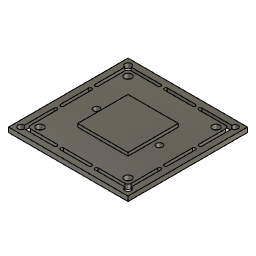
oat_guide_scope (Autodesk Fusion 360 archive; units mm, degrees)
design "ar0130"
Autodesk Fusion 360 part; units mm, degrees
sketch "Skizze1" plane through (0, 0, 0) normal (0, 0, 1) x (1, 0, 0)
  line L0 (-19, 19) -> (19, 19)
  line L1 (19, 19) -> (19, -19)
  line L2 (19, -19) -> (-19, -19)
  line L3 (-19, -19) -> (-19, 19)
  circle A0 centre (-14, 14) radius 1.175
  line L4 (0, 19) -> (0, -19) construction
  line L5 (-19, 0) -> (19, 0) construction
  circle A1 centre (14, 14) radius 1.175
  circle A2 centre (-14, -14) radius 1.175
  circle A3 centre (14, -14) radius 1.175
  circle A4 centre (-17, 17) radius 1
  circle A5 centre (17, 17) radius 1
  circle A6 centre (-17, -17) radius 1
  circle A7 centre (17, -17) radius 1
  circle A8 centre (-10, 0) radius 1
  circle A9 centre (10, 0) radius 1
  line L6 (-17, 16.5) -> (-6.5, 16.5) construction
  line L7 (-4.5, 16.5) -> (4.5, 16.5) construction
  line L8 (-4.5, 16) -> (4.5, 16)
  arc A10 (4.5, 16) -> (4.5, 17) centre (4.5, 16.5) ccw
  line L9 (4.5, 17) -> (-4.5, 17)
  arc A11 (-4.5, 17) -> (-4.5, 16) centre (-4.5, 16.5) ccw
  line L10 (-4.5, 16.5) -> (4.5, 16.5) construction
  line L11 (-6.5, 17) -> (-17, 17)
  arc A12 (-17, 17) -> (-17, 16) centre (-17, 16.5) ccw
  line L12 (-17, 16) -> (-6.5, 16)
  arc A13 (-6.5, 16) -> (-6.5, 17) centre (-6.5, 16.5) ccw
  line L13 (-6.5, 16.5) -> (-17, 16.5) construction
  line L14 (-19, 19) -> (19, -19) construction
  line L15 (6.5, 17) -> (17, 17)
  arc A14 (17, 16) -> (17, 17) centre (17, 16.5) ccw
  arc A15 (6.5, 17) -> (6.5, 16) centre (6.5, 16.5) ccw
  line L16 (17, 16) -> (6.5, 16)
  line L17 (-6.5, -17) -> (-17, -17)
  arc A16 (-17, -16) -> (-17, -17) centre (-17, -16.5) ccw
  arc A17 (-6.5, -17) -> (-6.5, -16) centre (-6.5, -16.5) ccw
  line L18 (4.5, -17) -> (-4.5, -17)
  arc A18 (-4.5, -16) -> (-4.5, -17) centre (-4.5, -16.5) ccw
  arc A19 (4.5, -17) -> (4.5, -16) centre (4.5, -16.5) ccw
  arc A20 (6.5, -16) -> (6.5, -17) centre (6.5, -16.5) ccw
  line L19 (6.5, -17) -> (17, -17)
  arc A21 (17, -17) -> (17, -16) centre (17, -16.5) ccw
  line L20 (17, -16) -> (6.5, -16)
  line L21 (-4.5, -16) -> (4.5, -16)
  line L22 (-17, -16) -> (-6.5, -16)
  line L23 (-17, -4.5) -> (-17, 4.5)
  arc A22 (-16, 4.5) -> (-17, 4.5) centre (-16.5, 4.5) ccw
  arc A23 (-17, -4.5) -> (-16, -4.5) centre (-16.5, -4.5) ccw
  line L24 (-16, 4.5) -> (-16, -4.5)
  arc A24 (17, 4.5) -> (16, 4.5) centre (16.5, 4.5) ccw
  line L25 (16, 4.5) -> (16, -4.5)
  arc A25 (16, -4.5) -> (17, -4.5) centre (16.5, -4.5) ccw
  line L26 (17, -4.5) -> (17, 4.5)
  line L27 (-17, 6.5) -> (-17, 17)
  arc A26 (-16, 17) -> (-17, 17) centre (-16.5, 17) ccw
  arc A27 (-17, 6.5) -> (-16, 6.5) centre (-16.5, 6.5) ccw
  line L28 (-16, 17) -> (-16, 6.5)
  arc A28 (-16, -6.5) -> (-17, -6.5) centre (-16.5, -6.5) ccw
  line L29 (-17, -6.5) -> (-17, -17)
  arc A29 (-17, -17) -> (-16, -17) centre (-16.5, -17) ccw
  line L30 (-16, -17) -> (-16, -6.5)
  arc A30 (17, 17) -> (16, 17) centre (16.5, 17) ccw
  line L31 (16, 17) -> (16, 6.5)
  arc A31 (16, 6.5) -> (17, 6.5) centre (16.5, 6.5) ccw
  line L32 (17, 6.5) -> (17, 17)
  line L33 (16, -17) -> (16, -6.5)
  arc A32 (17, -6.5) -> (16, -6.5) centre (16.5, -6.5) ccw
  arc A33 (16, -17) -> (17, -17) centre (16.5, -17) ccw
  line L34 (17, -6.5) -> (17, -17)
  dimension "d1" = 38
  dimension "d2" = 38
  dimension "d3" = 2.35
  dimension "d6" = 28
  dimension "d7" = 28
  dimension "d8" = 2
  dimension "d9" = 34
  dimension "d10" = 34
  dimension "d17" = 2
  dimension "d18" = 20
  dimension "d20" = 9
  dimension "d21" = 1
  dimension "d22" = 2
  dimension "d23" = 2.5
  dimension "d24" = 1
  dimension "d25" = 2
  constraint horizontal L0
  constraint vertical L1
  constraint horizontal L2
  constraint vertical L3
  constraint midpoint L0 L4.start
  constraint midpoint L2 L4.end
  constraint midpoint L3 L5.start
  constraint midpoint L1 L5.end
  constraint midpoint L5 origin
  constraint symmetric A0 L4 A1
  constraint symmetric A0 L5 A2
  constraint symmetric L5 A1 A3
  constraint symmetric L4 A4 A5
  constraint symmetric L5 A4 A6
  constraint symmetric L5 A5 A7
  constraint coincident L5 A8.centre
  constraint symmetric L4 A8 A9
  constraint horizontal L6
  constraint perpendicular L4 L7
  constraint symmetric L4 L7.start L7.end
  constraint tangent L8 A10
  constraint tangent A10 L9
  constraint parallel L8 L9
  constraint tangent L9 A11
  constraint tangent L8 A11
  constraint coincident L7.end A10.centre
  constraint parallel L7 L10
  constraint coincident L7.start A11.centre
  constraint tangent L11 A12
  constraint tangent A12 L12
  constraint parallel L11 L12
  constraint tangent L12 A13
  constraint tangent L11 A13
  constraint coincident L6.start A12.centre
  constraint parallel L6 L13
  constraint coincident L6.end A13.centre
  constraint collinear L7 L13
  constraint symmetric L4 L11.start L15.start
  constraint symmetric L4 A4.centre A5.centre
  constraint symmetric L4 A12.end A14.start
  constraint symmetric L4 L12.end A15.end
  constraint symmetric L4 A12 A14
  constraint symmetric L4 A13 A15
  constraint symmetric L5 L8.start A18.start
  constraint symmetric L5 L8.end A19.end
  constraint symmetric L5 A10.end L18.start
  constraint symmetric L5 L9.end L18.end
  constraint symmetric L5 A10 A19
  constraint symmetric L5 A11 A18
  constraint symmetric L5 L11.start L17.start
  constraint symmetric L5 A4.centre A6.centre
  constraint symmetric L5 A12.end A16.start
  constraint symmetric L5 L12.end A17.end
  constraint symmetric L5 A12 A16
  constraint symmetric L5 A13 A17
  constraint symmetric L5 L15.start A20.end
  constraint symmetric L5 A5.centre A7.centre
  constraint symmetric L5 A14.start A21.end
  constraint symmetric L5 A14 A21
  constraint symmetric L5 A15.end A20.start
  constraint symmetric L5 A15 A20
  constraint symmetric L8.start L14 A22.start
  constraint symmetric L8.end L14 A23.end
  constraint symmetric A10.end L14 L23.start
  constraint symmetric L9.end L14 L23.end
  constraint symmetric A10 L14 A23
  constraint symmetric A11 L14 A22
  constraint symmetric L11.start L14 L27.start
  constraint symmetric A4.centre L14 L11.end
  constraint symmetric A12.end L14 A26.start
  constraint symmetric L12.end L14 A27.end
  constraint symmetric A12 L14 A26
  constraint symmetric A13 L14 A27
  constraint symmetric L14 L15.start A28.end
  constraint symmetric L14 A5.centre A6.centre
  constraint symmetric L14 A14.start A29.end
  constraint symmetric L14 A14 A29
  constraint symmetric L14 A15.end A28.start
  constraint symmetric L14 A15 A28
  constraint symmetric L14 L17.start A31.end
  constraint symmetric L14 A6.centre A5.centre
  constraint symmetric L14 A16.start A30.end
  constraint symmetric L14 A16 A30
  constraint symmetric L14 A17.end L31.end
  constraint symmetric L14 A17 A31
  constraint symmetric L14 L18.start A25.end
  constraint symmetric L14 L18.end A24.start
  constraint symmetric L14 A18.start A24.end
  constraint symmetric L14 A18 A24
  constraint symmetric L14 A19.end L25.end
  constraint symmetric L14 A19 A25
  constraint symmetric L14 A20.end A32.start
  constraint symmetric L14 A20.start L33.end
  constraint symmetric L14 A20 A32
  constraint symmetric L14 A7.centre L19.end
  constraint symmetric L14 A21.end L33.start
  constraint symmetric L14 A21 A33
  measures "d1" distance of L0.start L0.end
  measures "d2" distance of L0.start L2.end
  measures "d3" diameter of A0
  measures "d6" distance of A0.centre A1.centre
  measures "d7" distance of A0.centre A2.centre
  measures "d8" diameter of A4
  measures "d9" distance of A4.centre A5.centre
  measures "d10" distance of A4.centre A6.centre
  measures "d17" diameter of A8
  measures "d18" distance of A8.centre A9.centre
  measures "d20" distance of L7.start L7.end
  measures "d21" diameter of A10
  measures "d22" distance of L6.end L7.start
  measures "d23" distance of L0 L7.end
  measures "d24" diameter of A12
  measures "d25" distance of L3 L6.start
extrude "Extrusion1" add sketch "Skizze1" along normal blind 1.5
fillet "Abrundung1" radius 1 4 edges at (-16, -16, 0.75) (16, -16, 0.75) (16, 16, 0.75) (-16, 16, 0.75)
sketch "Skizze2" plane through (0, 0, 1.5) normal (0, 0, 1) x (-1, 0, 0)
  circle A0 centre (14, -14) radius 1.175
  circle A1 centre (-14, 14) radius 1.175
  circle A2 centre (14, 14) radius 1.175
  circle A3 centre (-14, -14) radius 1.175
  line L0 (19, 19) -> (-19, 19)
  line L1 (-19, 19) -> (-19, -19)
  line L2 (-19, -19) -> (19, -19)
  line L3 (19, -19) -> (19, 19)
  line L4 (8, -8) -> (-8, -8)
  line L5 (-8, -8) -> (-8, 8)
  line L6 (-8, 8) -> (8, 8)
  line L7 (8, 8) -> (8, -8)
  line L8 (0, -19) -> (0, 19) construction
  line L9 (19, 0) -> (-19, 0) construction
  circle A4 centre (10, 0) radius 1
  circle A5 centre (-10, 0) radius 1
  line L10 (-17, -4.5) -> (-17, 4.5)
  arc A6 (-16, 4.5) -> (-17, 4.5) centre (-16.5, 4.5) ccw
  line L11 (-16, 4.5) -> (-16, -4.5)
  arc A7 (-17, -4.5) -> (-16, -4.5) centre (-16.5, -4.5) ccw
  line L12 (-6.5, 16) -> (-15, 16)
  line L13 (-16, 15) -> (-16, 6.5)
  arc A8 (-17, 6.5) -> (-16, 6.5) centre (-16.5, 6.5) ccw
  line L14 (-17, 6.5) -> (-17, 16)
  arc A9 (-16, 17) -> (-17, 16) centre (-17, 17) ccw
  line L15 (-16, 17) -> (-6.5, 17)
  arc A10 (-6.5, 16) -> (-6.5, 17) centre (-6.5, 16.5) ccw
  arc A11 (-4.5, 17) -> (-4.5, 16) centre (-4.5, 16.5) ccw
  line L16 (-4.5, 17) -> (4.5, 17)
  arc A12 (4.5, 16) -> (4.5, 17) centre (4.5, 16.5) ccw
  line L17 (4.5, 16) -> (-4.5, 16)
  line L18 (-16, -6.5) -> (-16, -15)
  line L19 (-15, -16) -> (-6.5, -16)
  arc A13 (-6.5, -17) -> (-6.5, -16) centre (-6.5, -16.5) ccw
  line L20 (-6.5, -17) -> (-16, -17)
  arc A14 (-17, -16) -> (-16, -17) centre (-17, -17) ccw
  line L21 (-17, -16) -> (-17, -6.5)
  arc A15 (-16, -6.5) -> (-17, -6.5) centre (-16.5, -6.5) ccw
  line L22 (16, 6.5) -> (16, 15)
  line L23 (15, 16) -> (6.5, 16)
  arc A16 (6.5, 17) -> (6.5, 16) centre (6.5, 16.5) ccw
  line L24 (6.5, 17) -> (16, 17)
  arc A17 (17, 16) -> (16, 17) centre (17, 17) ccw
  line L25 (17, 16) -> (17, 6.5)
  arc A18 (16, 6.5) -> (17, 6.5) centre (16.5, 6.5) ccw
  arc A19 (17, 4.5) -> (16, 4.5) centre (16.5, 4.5) ccw
  line L26 (17, 4.5) -> (17, -4.5)
  arc A20 (16, -4.5) -> (17, -4.5) centre (16.5, -4.5) ccw
  line L27 (16, -4.5) -> (16, 4.5)
  arc A21 (4.5, -17) -> (4.5, -16) centre (4.5, -16.5) ccw
  line L28 (4.5, -17) -> (-4.5, -17)
  arc A22 (-4.5, -16) -> (-4.5, -17) centre (-4.5, -16.5) ccw
  line L29 (-4.5, -16) -> (4.5, -16)
  line L30 (6.5, -16) -> (15, -16)
  line L31 (16, -15) -> (16, -6.5)
  arc A23 (17, -6.5) -> (16, -6.5) centre (16.5, -6.5) ccw
  line L32 (17, -6.5) -> (17, -16)
  arc A24 (16, -17) -> (17, -16) centre (17, -17) ccw
  line L33 (16, -17) -> (6.5, -17)
  arc A25 (6.5, -16) -> (6.5, -17) centre (6.5, -16.5) ccw
  arc A26 (15, -16) -> (16, -15) centre (15, -15) ccw
  arc A27 (-16, -15) -> (-15, -16) centre (-15, -15) ccw
  arc A28 (-15, 16) -> (-16, 15) centre (-15, 15) ccw
  arc A29 (16, 15) -> (15, 16) centre (15, 15) ccw
  dimension "d13" = 16
  dimension "d14" = 16
  constraint horizontal L4
  constraint vertical L5
  constraint horizontal L6
  constraint vertical L7
  constraint midpoint L2 L8.start
  constraint midpoint L0 L8.end
  constraint midpoint L3 L9.start
  constraint midpoint L1 L9.end
  constraint symmetric L4 L6 L9
  constraint symmetric L5 L7 L8
  measures "d13" distance of L4.start L4.end
  measures "d14" distance of L4.start L6.end
extrude "Extrusion2" add sketch "Skizze2" along normal blind 1 contours L4 L5 L6 L7
sketch "Skizze3" plane through (0, 0, 0) normal (0, 0, -1) x (1, 0, 0)
  circle A0 centre (-14, 14) radius 1.175
  arc A1 (-4.5, -16) -> (-4.5, -17) centre (-4.5, -16.5) ccw
  line L0 (-4.5, -16) -> (4.5, -16)
  arc A2 (4.5, -17) -> (4.5, -16) centre (4.5, -16.5) ccw
  line L1 (4.5, -17) -> (-4.5, -17)
  circle A3 centre (-14, -14) radius 1.175
  circle A4 centre (14, -14) radius 1.175
  line L2 (-16, 15) -> (-16, 6.5)
  arc A5 (-17, 6.5) -> (-16, 6.5) centre (-16.5, 6.5) ccw
  line L3 (-17, 6.5) -> (-17, 16)
  arc A6 (-16, 17) -> (-17, 16) centre (-17, 17) ccw
  line L4 (-16, 17) -> (-6.5, 17)
  arc A7 (-6.5, 16) -> (-6.5, 17) centre (-6.5, 16.5) ccw
  line L5 (-6.5, 16) -> (-15, 16)
  circle A8 centre (-10, 0) radius 1
  line L6 (-15, -16) -> (-6.5, -16)
  arc A9 (-6.5, -17) -> (-6.5, -16) centre (-6.5, -16.5) ccw
  line L7 (-6.5, -17) -> (-16, -17)
  arc A10 (-17, -16) -> (-16, -17) centre (-17, -17) ccw
  line L8 (-17, -16) -> (-17, -6.5)
  arc A11 (-16, -6.5) -> (-17, -6.5) centre (-16.5, -6.5) ccw
  line L9 (-16, -6.5) -> (-16, -15)
  arc A12 (-16, 4.5) -> (-17, 4.5) centre (-16.5, 4.5) ccw
  line L10 (-16, 4.5) -> (-16, -4.5)
  arc A13 (-17, -4.5) -> (-16, -4.5) centre (-16.5, -4.5) ccw
  line L11 (-17, -4.5) -> (-17, 4.5)
  line L12 (15, 16) -> (6.5, 16)
  arc A14 (6.5, 17) -> (6.5, 16) centre (6.5, 16.5) ccw
  line L13 (6.5, 17) -> (16, 17)
  arc A15 (17, 16) -> (16, 17) centre (17, 17) ccw
  line L14 (17, 16) -> (17, 6.5)
  arc A16 (16, 6.5) -> (17, 6.5) centre (16.5, 6.5) ccw
  line L15 (16, 6.5) -> (16, 15)
  line L16 (16, -15) -> (16, -6.5)
  arc A17 (17, -6.5) -> (16, -6.5) centre (16.5, -6.5) ccw
  line L17 (17, -6.5) -> (17, -16)
  arc A18 (16, -17) -> (17, -16) centre (17, -17) ccw
  line L18 (16, -17) -> (6.5, -17)
  arc A19 (6.5, -16) -> (6.5, -17) centre (6.5, -16.5) ccw
  line L19 (6.5, -16) -> (15, -16)
  arc A20 (4.5, 16) -> (4.5, 17) centre (4.5, 16.5) ccw
  line L20 (4.5, 16) -> (-4.5, 16)
  arc A21 (-4.5, 17) -> (-4.5, 16) centre (-4.5, 16.5) ccw
  line L21 (-4.5, 17) -> (4.5, 17)
  circle A22 centre (14, 14) radius 1.175
  line L22 (17, 4.5) -> (17, -4.5)
  arc A23 (16, -4.5) -> (17, -4.5) centre (16.5, -4.5) ccw
  line L23 (16, -4.5) -> (16, 4.5)
  arc A24 (17, 4.5) -> (16, 4.5) centre (16.5, 4.5) ccw
  circle A25 centre (10, 0) radius 1
  line L24 (19, 19) -> (-19, 19)
  line L25 (-19, 19) -> (-19, -19)
  line L26 (-19, -19) -> (19, -19)
  line L27 (19, -19) -> (19, 19)
  arc A26 (-15, 16) -> (-16, 15) centre (-15, 15) ccw
  arc A27 (-16, -15) -> (-15, -16) centre (-15, -15) ccw
  arc A28 (16, 15) -> (15, 16) centre (15, 15) ccw
  arc A29 (15, -16) -> (16, -15) centre (15, -15) ccw
